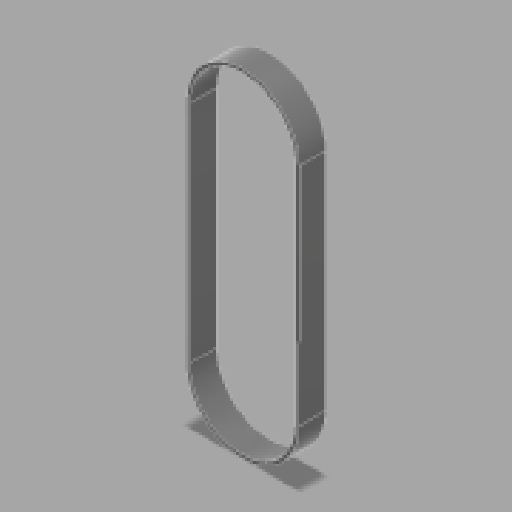
# Autodesk Inventor part: Ремень
Saved by Autodesk Inventor 2025 (Build 290162000, 162)
## iProperties
Created: 2025-04-08
Part Number: Ремень
Material: Типовые
Document SubType Name: Modeling
Designer: Artem Sannikov
Density: 1 g/cm^3
Appearance: Гладкая — черная
Author: Artem Sannikov
Autodesk Inventor part; units mm, degrees
ref_plane "YZ Plane" through (0, 0, 0) normal (1, 0, 0) x (0, 1, 0)
ref_plane "XZ Plane" through (0, 0, 0) normal (0, 1, 0) x (-1, 0, 0)
ref_plane "XY Plane" through (0, 0, 0) normal (0, 0, 1) x (1, 0, 0)
sketch "Эскиз1" plane through (0, 0, 0) normal (0, 0, 1) x (1, 0, 0)
  spline S0 degree 3 number of poles 571 construction
  circle A0 centre (0, 0) radius 12.4728
  circle A1 centre (0, 0) radius 11.6873
  spline S1 degree 3 number of poles 571 construction
  circle A2 centre (0.0593, 50) radius 3.05 construction
  circle A3 centre (0.0593, 50) radius 12.4622
  circle A4 centre (0.0593, 50) radius 11.6915
  line L0 (12.5215, 49.9878) -> (12.4728, -0.0121)
  line L1 (-12.4028, 50.0174) -> (-12.4728, 0.0175)
  line L2 (-11.6322, 50.0129) -> (-11.6873, 0.0129)
  line L3 (-11.6921, -4.3435) -> (-11.689, -1.4984)
  line L4 (11.7508, 49.9851) -> (11.6873, -0.0148)
  line L5 (0, 0) -> (-30.3964, 0.0335) construction
  point P0 (-23.5791, 58.2576)
  point P1 (2.2116, 51.4848)
  point P2 (12.4728, 0)
  dimension "d0" = 24.9244
  dimension "d1" = 24.9457
  dimension "d2" = 23.383
  dimension "d3" = 23.3746
  dimension "d6" = 50
  constraints: 12 end point, 10 tangent, 9 point on circle, 5 centre point, 4 coincident, 1 perpendicular, 1 other
  measures "d0" diameter of A3
  measures "d1" diameter of A0
  measures "d2" diameter of A4
  measures "d3" diameter of A1
  measures "d6" distance from line of L5 A2.centre
extrude "Выдавливание1" add sketch "Эскиз1" along normal blind 6 contours A0 L2 A1 L4 | L1 A3 L2 A0 | A3 L4 A4 L2 | L4 A3 L0 A0 picked at (-11.8082, -1.4117) picked at (12.144, 50.9937)
